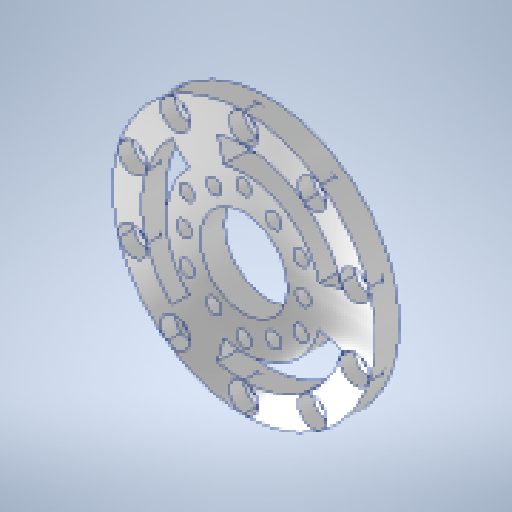
# Autodesk Inventor part: link2part2
Saved by Autodesk Inventor 2024 (Build 280153000, 153)
## iProperties
Created: 2025-02-08
Part Number: link2part2
Material: アルミニウム 6061
Document SubType Name: Modeling
Designer: tanoue_kota
Density: 2.7 g/cm^3
Appearance: アルミニウム - フラット
Mass: 17.6775 g
Surface Area: 63.6498 cm^2
Volume: 6.54724 cm^3
Author: tanoue_kota
Autodesk Inventor part; units mm, degrees
ref_plane "YZ Plane" through (0, 0, 0) normal (1, 0, 0) x (0, 1, 0)
ref_plane "XZ Plane" through (0, 0, 0) normal (0, 1, 0) x (-1, 0, 0)
ref_plane "XY Plane" through (0, 0, 0) normal (0, 0, 1) x (1, 0, 0)
sketch "スケッチ1" plane through (0, 0, 0) normal (0, 0, 1) x (1, 0, 0)
  circle A0 centre (0, 0) radius 13.5
  circle A1 centre (0, 0) radius 27
  dimension "d0" = 27
  dimension "d1" = 54
  constraints: 2 centre point, 2 coincident
  measures "d0" diameter of A0
  measures "d1" diameter of A1
sketch "スケッチ1 outline for 押し出し1" plane through (0, 0, 0) normal (0, 0, 1) x (1, 0, 0)
  circle A0 centre (0, 0) radius 27
extrude "押し出し1" add sketch "スケッチ1 outline for 押し出し1" along normal blind 5
sketch "スケッチ2" plane through (0, 0, 5) normal (0, 0, 1) x (1, 0, 0)
  circle A0 centre (0, 0) radius 13.5
  circle A1 centre (0, 0) radius 12.23
  line L0 (0, 13.5) -> (0, 0)
  line L1 (0, 0) -> (6.115, 10.591491)
  point P0 (-11.691343, 6.75)
  point P1 (-11.691343, -6.75)
  point P2 (0, -13.5)
  point P3 (11.691343, -6.75)
  point P4 (11.691343, 6.75)
  point P5 (6.115, 10.591491)
  point P6 (-6.115, 10.591491)
  point P7 (-12.23, 0)
  point P8 (-6.115, -10.591491)
  point P9 (6.115, -10.591491)
  point P10 (12.23, 0)
  dimension "d4" = 27
  dimension "d9" = 24.46
  dimension "d7" = 360
  dimension "d10" = 30
  dimension "d13" = 360
  constraints: 4 end point, 3 coincident, 1 vertical, 1 vertical alignment, 19 other
  measures "d10" angle of L0 L1
hole "穴1" at (0, 13.5, 5) at (-11.691343, 6.75, 5) at (-11.691343, -6.75, 5) at (0, -13.5, 5) at (11.691343, -6.75, 5) at (11.691343, 6.75, 5) at (6.115, 10.591491, 5) at (-6.115, 10.591491, 5) at (-12.23, 0, 5) at (-6.115, -10.591491, 5) at (6.115, -10.591491, 5) at (12.23, 0, 5) direction (0, 0, -1) diameter 3.2 end through all
sketch "スケッチ3" plane through (0, 0, 0) normal (0, 0, -1) x (-1, 0, 0)
  line L0 (0, 0) -> (0, -24)
  point P0 (14.106846, -19.416408)
  point P1 (22.825356, -7.416408)
  point P2 (22.825356, 7.416408)
  point P3 (14.106846, 19.416408)
  point P4 (0, 24)
  point P5 (-14.106846, 19.416408)
  point P6 (-22.825356, 7.416408)
  point P7 (-22.825356, -7.416408)
  point P8 (-14.106846, -19.416408)
  dimension "d65" = 24
  dimension "d68" = 360
  constraints: 2 coincident, 2 end point, 1 vertical, 11 other
  measures "d65" distance of L0.start L0.end
hole "穴2" at (-14.106846, -19.416408, 0) at (-22.825356, -7.416408, 0) at (-22.825356, 7.416408, 0) at (-14.106846, 19.416408, 0) at (0, 24, 0) at (14.106846, 19.416408, 0) at (22.825356, 7.416408, 0) at (22.825356, -7.416408, 0) at (14.106846, -19.416408, 0) at (0, -24, 0) direction (0, 0, 1) diameter 3.2 depth 20 tip angle 118
sketch "スケッチ4" plane through (0, 0, 0) normal (0, 0, -1) x (-1, 0, 0)
  circle A0 centre (0, 0) radius 9
  circle A1 centre (0, 0) radius 21
  circle A2 centre (0, 0) radius 16
  line L0 (-21, 0) -> (0, 0)
  line L1 (0, 0) -> (-20.284442, 5.4352)
  line L2 (0, 0) -> (-20.284442, -5.4352)
  line L3 (0, 0) -> (14.849242, -14.849242)
  line L4 (0, 0) -> (5.4352, -20.284442)
  line L5 (0, 0) -> (5.4352, 20.284442)
  line L6 (0, 0) -> (14.849242, 14.849242)
  point P0 (14.849242, 14.849242)
  point P1 (11.313708, 11.313708)
  point P2 (11.313708, -11.313708)
  point P3 (14.849242, -14.849242)
  point P4 (4.141105, 15.454813)
  point P5 (5.4352, 20.284442)
  point P6 (-15.454813, 4.141105)
  point P7 (5.4352, -20.284442)
  point P8 (4.141105, -15.454813)
  point P9 (-15.454813, -4.141105)
  point P10 (-20.284442, -5.4352)
  dimension "d39" = 18
  dimension "d40" = 42
  dimension "d41" = 32
  dimension "d42" = 15
  dimension "d45" = 360
  constraints: 14 end point, 3 centre point, 3 coincident, 2 point on circle, 1 horizontal, 1 symmetric about line, 16 other
  measures "d39" diameter of A0
  measures "d40" diameter of A1
  measures "d41" diameter of A2
  measures "d42" angle of L0 L1
sketch "スケッチ4 outline for 押し出し2" plane through (0, 0, 0) normal (0, 0, -1) x (-1, 0, 0)
  line L0 (14.849242, 14.849242) -> (11.313708, 11.313708)
  arc A0 (14.849242, -14.849242) -> (14.849242, 14.849242) centre (0, 0) ccw
  line L1 (11.313708, -11.313708) -> (14.849242, -14.849242)
  arc A1 (11.313708, 11.313708) -> (11.313708, -11.313708) centre (0, 0) cw
  line L2 (4.141105, 15.454813) -> (5.4352, 20.284442)
  arc A2 (-15.454813, 4.141105) -> (4.141105, 15.454813) centre (0, 0) cw
  line L3 (-20.284442, 5.4352) -> (-15.454813, 4.141105)
  arc A3 (5.4352, 20.284442) -> (-20.284442, 5.4352) centre (0, 0) ccw
  line L4 (5.4352, -20.284442) -> (4.141105, -15.454813)
  arc A4 (-20.284442, -5.4352) -> (5.4352, -20.284442) centre (0, 0) ccw
  line L5 (-15.454813, -4.141105) -> (-20.284442, -5.4352)
  arc A5 (4.141105, -15.454813) -> (-15.454813, -4.141105) centre (0, 0) cw
  circle A6 centre (0, 0) radius 9
extrude "押し出し2" cut sketch "スケッチ4 outline for 押し出し2" against normal blind 5
sketch "スケッチ6" plane through (0, 0, 5) normal (0, 0, 1) x (1, 0, 0)
  circle A0 centre (0, -24) radius 1.6
  circle A1 centre (0, -24) radius 3
  circle A2 centre (14.106846, -19.416408) radius 3
  circle A3 centre (22.825356, -7.416408) radius 3
  circle A4 centre (22.825356, 7.416408) radius 3
  circle A5 centre (14.106846, 19.416408) radius 3
  circle A6 centre (0, 24) radius 3
  circle A7 centre (-14.106846, 19.416408) radius 3
  circle A8 centre (-22.825356, 7.416408) radius 3
  circle A9 centre (-22.825356, -7.416408) radius 3
  circle A10 centre (-14.106846, -19.416408) radius 3
  point P0 (0, 0)
  dimension "d70" = 6
  dimension "d73" = 360
  constraints: 10 centre point, 1 coincident, 21 other
  measures "d70" diameter of A1
sketch "スケッチ6 outline for 押し出し4" plane through (0, 0, 5) normal (0, 0, 1) x (1, 0, 0)
  circle A0 centre (14.106846, -19.416408) radius 3
  circle A1 centre (22.825356, -7.416408) radius 3
  circle A2 centre (22.825356, 7.416408) radius 3
  circle A3 centre (14.106846, 19.416408) radius 3
  circle A4 centre (0, 24) radius 3
  circle A5 centre (-14.106846, 19.416408) radius 3
  circle A6 centre (-22.825356, 7.416408) radius 3
  circle A7 centre (-22.825356, -7.416408) radius 3
  circle A8 centre (-14.106846, -19.416408) radius 3
  circle A9 centre (0, -24) radius 3
extrude "押し出し4" cut sketch "スケッチ6 outline for 押し出し4" against normal blind 3
